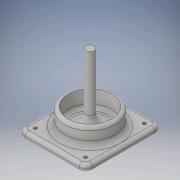
# Autodesk Inventor part: Upper_part
Saved by Autodesk Inventor 2016 (Build 200138000, 138)
## iProperties
Created: 2018-11-02
Part Number: Upper_part
Material: Generic
Document SubType Name: Modeling
Designer: attila
Density: 1 g/cm^3
Appearance: Default
Author: attila
Autodesk Inventor part; units mm, degrees
ref_plane "YZ Plane" through (0, 0, 0) normal (1, 0, 0) x (0, 1, 0)
ref_plane "XZ Plane" through (0, 0, 0) normal (0, 1, 0) x (-1, 0, 0)
ref_plane "XY Plane" through (0, 0, 0) normal (0, 0, 1) x (1, 0, 0)
sketch "Sketch1" plane through (0, 0, 0) normal (0, 1, 0) x (-1, 0, 0)
  line L0 (20, 22.5) -> (-20, 22.5)
  line L1 (-20, 22.5) -> (-20, -22.5)
  line L2 (-20, -22.5) -> (20, -22.5)
  line L3 (20, -22.5) -> (20, 22.5)
  point P0 (0, 0)
  point P1 (-20, 0)
  point P2 (20, 0)
  point P3 (0, 22.5)
  point P4 (0, -22.5)
  dimension "d2" = 45
  dimension "d3" = 40
  constraints: 8 end point, 4 midpoint, 2 horizontal alignment, 2 parallel, 2 vertical alignment, 1 horizontal, 1 perpendicular
  measures "d2" distance of L0.end L1.end
  measures "d3" distance of L1.end L2.end
extrude "Extrusion1" add sketch "Sketch1" along normal blind 3
sketch "Sketch2" plane through (0, 3, 0) normal (0, 1, 0) x (1, 0, 0)
  circle A0 centre (0, 0) radius 2.5
  dimension "d4" = 5
  constraints: 1 centre point, 1 coincident
  measures "d4" diameter of A0
extrude "Extrusion2" add sketch "Sketch2" along normal blind 40
fillet "Fillet1" radius 7 1 edges at (-2.5, 3, 0)
sketch "Sketch3" plane through (0, 3, 0) normal (0, 1, 0) x (1, 0, 0)
  circle A0 centre (0, 0) radius 13
  circle A1 centre (0, 0) radius 15
  dimension "d8" = 26
  dimension "d9" = 30
  constraints: 2 centre point, 2 coincident
  measures "d8" diameter of A0
  measures "d9" diameter of A1
extrude "Extrusion3" add sketch "Sketch3" along normal blind 10
sketch "Sketch4" plane through (0, 3, 0) normal (0, 1, 0) x (1, 0, 0)
  line L0 (20, 22.5) -> (-20, 22.5) projected
  line L1 (20, -22.5) -> (20, 22.5) projected
  line L2 (-20, -22.5) -> (20, -22.5) projected
  line L3 (-20, 22.5) -> (-20, -22.5) projected
  point P0 (0, 0)
  point P1 (15, -17.5)
  point P2 (15, 17.5)
  point P3 (-15, 17.5)
  point P4 (-15, -17.5)
  dimension "d12" = 5
  dimension "d13" = 5
  dimension "d14" = 5
  dimension "d15" = 5
  dimension "d16" = 5
  dimension "d17" = 5
  dimension "d18" = 5
  dimension "d19" = 5
  measures "d12" distance from line of L0 point (15, 17.5)
  measures "d13" distance from line of L1 point (15, 17.5)
  measures "d14" distance from line of L1 point (15, -17.5)
  measures "d15" distance from line of L2 point (15, -17.5)
  measures "d16" distance from line of L3 point (-15, -17.5)
  measures "d17" distance from line of L2 point (-15, -17.5)
  measures "d18" distance from line of L3 point (-15, 17.5)
  measures "d19" distance from line of L0 point (-15, 17.5)
hole "Hole1" at (15, 3, 17.5) at (15, 3, -17.5) at (-15, 3, -17.5) at (-15, 3, 17.5) direction (0, -1, 0) diameter 2 end through all
fillet "Fillet2" radius 3 1 edges at (-15, 3, 0)
fillet "Fillet3" radius 2 1 edges at (-13, 3, 0)
fillet "Fillet4" radius 4 4 edges at (20, 1.5, 22.5) (20, 1.5, -22.5) (-20, 1.5, 22.5) (-20, 1.5, -22.5)
fillet "Fillet5" radius 2 8 edges at (-18.8284, 3, 21.3284) (0, 3, 22.5) (18.8284, 3, 21.3284) (20, 3, 0) (18.8284, 3, -21.3284) (0, 3, -22.5) (-18.8284, 3, -21.3284) (-20, 3, 0)
fillet "Fillet6" radius 2 1 edges at (-15, 13, 0)
equation "\"d13\" = d12"
equation "\"d14\" = d15"
equation "\"d17\" = d16"
equation "\"d19\" = d18"
body "Solid1"
